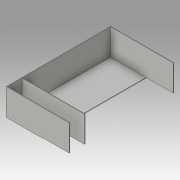
# Autodesk Inventor part: Collector Base
Saved by Autodesk Inventor 2016 (Build 200138000, 138)
## iProperties
Created: 2015-12-26
Part Number: Collector Base
Material: Generic
Document SubType Name: Modeling
Designer: Delta
Density: 1 g/cm^3
Appearance: Default
Author: Delta
Autodesk Inventor part; units mm, degrees
ref_plane "YZ Plane" through (0, 0, 0) normal (1, 0, 0) x (0, 1, 0)
ref_plane "XZ Plane" through (0, 0, 0) normal (0, 1, 0) x (-1, 0, 0)
ref_plane "XY Plane" through (0, 0, 0) normal (0, 0, 1) x (1, 0, 0)
sketch "Sketch1" plane through (0, 0, 0) normal (0, 1, 0) x (-1, 0, 0)
  point P0 (0, 0)
sketch "Sketch2" plane through (0, 0, 0) normal (0, 1, 0) x (-1, 0, 0)
  line L0 (0, 0) -> (104.775, 0)
  line L1 (104.775, 0) -> (104.775, -304.8)
  line L2 (104.775, -304.8) -> (0, -304.8)
  line L3 (0, -304.8) -> (0, 0)
  dimension "d0" = 104.775
  dimension "d1" = 304.8
  constraints: 8 end point, 2 parallel, 1 horizontal, 1 perpendicular
  measures "d0" distance of L1.end L2.end
  measures "d1" distance of L0.end L1.end
extrude "Extrusion1" add sketch "Sketch2" along normal blind 1.5875
sketch "Sketch3" plane through (0, 1.5875, 0) normal (0, 1, 0) x (1, 0, 0)
  line L0 (-104.775, 0) -> (0, 0) projected
  line L1 (-104.775, 0) -> (-103.1875, 0)
  line L2 (-103.1875, 0) -> (-103.1875, 304.8)
  line L3 (-104.775, 304.8) -> (-104.775, 0)
  line L4 (-104.775, 304.8) -> (-104.775, 0) projected
  line L5 (-104.775, 0) -> (79.375, 0)
  line L6 (79.375, 0) -> (79.375, 1.5875)
  line L7 (79.375, 1.5875) -> (-104.775, 1.5875)
  line L8 (-104.775, 1.5875) -> (-104.775, 0)
  line L9 (0, 304.8) -> (-104.775, 304.8) projected
  line L10 (-104.775, 304.8) -> (79.375, 304.8)
  line L11 (79.375, 304.8) -> (79.375, 303.2125)
  line L12 (79.375, 303.2125) -> (-104.775, 303.2125)
  line L13 (-104.775, 303.2125) -> (-104.775, 304.8)
  line L14 (-104.775, 304.8) -> (-103.1875, 304.8)
  line L15 (-103.1875, 304.8) -> (-103.1875, 0)
  line L16 (-103.1875, 0) -> (-104.775, 0)
  line L17 (-104.775, 0) -> (-104.775, 304.8)
  dimension "d6" = 184.15
  dimension "d7" = 1.5875
  dimension "d8" = 184.15
  dimension "d9" = 1.5875
  dimension "d10" = 1.5875
  dimension "d11" = 304.8
  constraints: 30 end point, 7 parallel, 4 horizontal, 4 perpendicular
  measures "d6" distance of L7.end L6.end
  measures "d7" distance of L6.end L5.end
  measures "d8" distance of L11.end L12.end
  measures "d9" distance of L10.end L11.end
  measures "d10" distance of L1.end L16.end
  measures "d11" distance of L14.end L1.end
extrude "Extrusion2" add sketch "Sketch3" along normal blind 76.2
sketch "Sketch4" plane through (-103.1875, 1.5875, -1.5875) normal (1, 0, 0) x (0, 0, -1)
  line L0 (-1.5875, -1.5875) -> (-1.5875, 0) construction
  line L1 (-1.5875, -1.5875) -> (42.8625, -1.5875) construction
  line L2 (303.2125, -1.5875) -> (-1.5875, -1.5875) construction
  line L3 (42.8625, -1.5875) -> (42.8625, 0) construction
  line L4 (0, 0) -> (301.625, 0) construction
  line L5 (0, 76.2) -> (301.625, 76.2) projected
  line L6 (42.8625, 0) -> (44.45, 0)
  line L7 (44.45, 0) -> (44.45, 76.2)
  line L8 (44.45, 76.2) -> (42.8625, 76.2)
  line L9 (42.8625, 76.2) -> (42.8625, 0)
  dimension "d14" = 44.45
  dimension "d15" = 1.5875
  constraints: 12 end point, 3 point on line, 2 parallel, 2 perpendicular, 1 horizontal
  measures "d14" distance of L0.start L1.end
  measures "d15" distance of L8.end L7.end
extrude "Extrusion3" add sketch "Sketch4" along normal blind 182.5625
body "Solid1"
